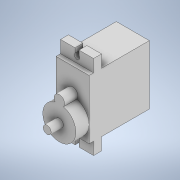
# Autodesk Inventor part: Сервопривод SG90
Saved by Autodesk Inventor 2020 (Build 240168000, 168)
## iProperties
Created: 2019-07-06
Part Number: Сервопривод SG90
Material: Типовые
Document SubType Name: Modeling
Designer: ivanc
Density: 1 g/cm^3
Appearance: По умолчанию
Author: ivanc
Autodesk Inventor part; units mm, degrees
ref_plane "YZ Plane" through (0, 0, 0) normal (1, 0, 0) x (0, 1, 0)
ref_plane "XZ Plane" through (0, 0, 0) normal (0, 1, 0) x (-1, 0, 0)
ref_plane "XY Plane" through (0, 0, 0) normal (0, 0, 1) x (1, 0, 0)
sketch "Эскиз2" plane through (0, 0, 0) normal (0, 0, 1) x (1, 0, 0)
  line L0 (0, 0) -> (12.5, 0)
  line L1 (12.5, 0) -> (12.5, 22.4)
  line L2 (12.5, 22.4) -> (0, 22.4)
  line L3 (0, 22.4) -> (0, 0)
  dimension "d0" = 12.5
  dimension "d1" = 22.4
  constraints: 8 end point, 2 parallel, 1 horizontal, 1 perpendicular
  measures "d0" distance of L2.end L1.end
  measures "d1" distance of L1.end L0.end
extrude "Выдавливание1" add sketch "Эскиз2" along normal blind 22.8
sketch "Эскиз3" plane through (0, 22.4, 0) normal (0, 1, 0) x (1, 0, 0)
  line L0 (12.5, 0) -> (0, 0) projected
  line L1 (12.5, 0) -> (12.5, -18.1)
  line L2 (12.5, 0) -> (12.5, -22.8) projected
  line L3 (0, 0) -> (0, -22.8) projected
  line L4 (12.5, -18.1) -> (0, -18.1)
  line L5 (0, -18.1) -> (0, -21.1)
  line L6 (0, -21.1) -> (12.5, -21.1)
  line L7 (12.5, -21.1) -> (12.5, -18.1)
  point P0 (12.5, -21.1)
  point P1 (0, -18.1)
  dimension "d4" = 18.1
  dimension "d5" = 3
  constraints: 10 end point, 2 parallel, 2 point on line, 1 horizontal, 1 perpendicular
  measures "d4" distance of L0.start L1.end
  measures "d5" distance of L5.end L4.end
extrude "Выдавливание2" add sketch "Эскиз3" along normal blind 4.7 contours L2 L6 L3 L4
sketch "Эскиз4" plane through (0, 0, 0) normal (0, -1, 0) x (1, 0, 0)
  line L0 (12.2114, 0) -> (12.5, 16.0974)
  line L1 (12.5, 0) -> (12.5, 22.8) projected
  line L2 (12.5, 21.1) -> (12.5, 18.1) projected
  line L3 (0, 18.1) -> (0, 21.1) projected
  line L4 (12.5, 18.1) -> (0, 18.1)
  line L5 (0, 18.1) -> (0, 21.1)
  line L6 (0, 21.1) -> (12.5, 21.1)
  line L7 (12.5, 21.1) -> (12.5, 18.1)
  point P0 (0, 0)
  point P1 (12.5, 21.1)
  point P2 (0, 18.1)
  dimension "d8" = 16.1
  dimension "d9" = 3
  constraints: 10 end point, 2 parallel, 1 horizontal, 1 perpendicular, 1 point on line
  measures "d8" distance of L0.start L0.end
  measures "d9" distance of L4.end L3.end
extrude "Выдавливание3" add sketch "Эскиз4" along normal blind 4.7
sketch "Эскиз5" plane through (0, 0, 21.1) normal (0, 0, 1) x (1, 0, 0)
  line L0 (0, -4.7) -> (12.5, -4.7) projected
  line L1 (6.25, -4.7) -> (6.25, -2.275)
  line L2 (12.5, 27.1) -> (0, 27.1) projected
  line L3 (6.25, 27.1) -> (6.25, 24.675)
  circle A0 centre (6.25, -2.275) radius 1
  circle A1 centre (6.25, 24.675) radius 1
  line L4 (6.25, -2.275) -> (7, -2.275)
  line L5 (7, -2.275) -> (7, -4.7)
  line L6 (7, -4.7) -> (6.25, -4.7)
  line L7 (6.25, -4.7) -> (6.25, -2.275)
  line L8 (6.25, -4.7) -> (5.5, -4.7)
  line L9 (5.5, -4.7) -> (5.5, -2.275)
  line L10 (5.5, -2.275) -> (6.25, -2.275)
  line L11 (6.25, -2.275) -> (6.25, -4.7)
  line L12 (6.25, 27.1) -> (7, 27.1)
  line L13 (7, 27.1) -> (7, 24.675)
  line L14 (7, 24.675) -> (6.25, 24.675)
  line L15 (6.25, 24.675) -> (6.25, 27.1)
  line L16 (6.25, 24.675) -> (5.5, 24.675)
  line L17 (5.5, 24.675) -> (5.5, 27.1)
  line L18 (5.5, 27.1) -> (6.25, 27.1)
  line L19 (6.25, 27.1) -> (6.25, 24.675)
  point P0 (0, 0)
  point P1 (5.5, 25.3364)
  point P2 (7, 25.3364)
  point P3 (5.5, -2.9364)
  point P4 (7, -2.9364)
  dimension "d12" = 2.425
  dimension "d13" = 2.425
  dimension "d14" = 2
  dimension "d15" = 2
  dimension "d16" = 0.75
  dimension "d17" = 0.75
  dimension "d18" = 0.75
  dimension "d19" = 0.75
  constraints: 36 end point, 8 parallel, 4 horizontal, 4 perpendicular, 2 centre point, 2 coincident, 2 midpoint, 2 point on line, 2 vertical
  measures "d12" distance of L1.start L1.end
  measures "d13" distance of L3.start L3.end
  measures "d14" diameter of A0
  measures "d15" diameter of A1
  measures "d16" distance of L5.end L6.end
  measures "d17" distance of L9.end L10.end
  measures "d18" distance of L13.end L14.end
  measures "d19" distance of L17.end L18.end
extrude "Выдавливание4" cut sketch "Эскиз5" against normal through all
sketch "Эскиз6" plane through (0, 0, 22.8) normal (0, 0, 1) x (1, 0, 0)
  line L0 (12.5, 0) -> (0, 0) projected
  line L1 (6.25, 0) -> (6.25, 6.25)
  circle A0 centre (6.25, 6.25) radius 6.25
  line L2 (6.25, 6.25) -> (6.25, 13.5)
  circle A1 centre (6.25, 13.5) radius 2
  point P0 (7.8448, 12.2931)
  dimension "d22" = 6.25
  dimension "d23" = 12.5
  dimension "d24" = 7.25
  dimension "d25" = 4
  constraints: 4 end point, 2 centre point, 2 coincident, 2 vertical, 1 midpoint
  measures "d22" distance of L1.start L1.end
  measures "d23" diameter of A0
  measures "d24" distance of L2.start L2.end
  measures "d25" diameter of A1
extrude "Выдавливание5" add sketch "Эскиз6" along normal blind 5
sketch "Эскиз7" plane through (0, 0, 27.8) normal (0, 0, 1) x (1, 0, 0)
  arc A0 (4.6552, 12.2931) -> (0, 6.25) centre (6.25, 6.25) ccw projected
  circle A1 centre (6.25, 6.25) radius 1.5
  point P0 (0, 0)
  dimension "d28" = 3
  constraints: 1 centre point, 1 coincident
  measures "d28" diameter of A1
extrude "Выдавливание6" add sketch "Эскиз7" along normal blind 4.6
